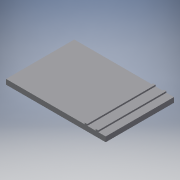
# Autodesk Inventor part: Zijkant 3
Saved by Autodesk Inventor 2018.3 (Build 223284000, 284)
## iProperties
Created: 2020-11-10
Part Number: Zijkant 3
Material: Generic
Document SubType Name: Modeling
Designer: daanv
Density: 1 g/cm^3
Appearance: Default
Author: daanv
Autodesk Inventor part; units mm, degrees
ref_plane "YZ Plane" through (0, 0, 0) normal (1, 0, 0) x (0, 1, 0)
ref_plane "XZ Plane" through (0, 0, 0) normal (0, 1, 0) x (-1, 0, 0)
ref_plane "XY Plane" through (0, 0, 0) normal (0, 0, 1) x (1, 0, 0)
sketch "Sketch1" plane through (0, 0, 0) normal (0, 0, 1) x (1, 0, 0)
  line L0 (0, 0) -> (20, 0)
  line L1 (20, 0) -> (20, 13.7)
  line L2 (20, 13.7) -> (0, 13.7)
  line L3 (0, 13.7) -> (0, 0)
  dimension "d0" = 20
  dimension "d1" = 13.7
  constraints: 8 end point, 2 parallel, 1 horizontal, 1 perpendicular
  measures "d0" distance of L2.end L1.end
  measures "d1" distance of L1.end L0.end
extrude "Extrusion1" add sketch "Sketch1" along normal blind 1
sketch "Sketch2" plane through (0, 0, 1) normal (0, 0, 1) x (1, 0, 0)
  line L0 (0, 0) -> (20, 0) projected
  line L1 (20, 13.7) -> (0, 13.7) projected
  line L2 (13.7, 13.7) -> (12.7, 13.7)
  line L3 (12.7, 13.7) -> (12.7, 0)
  line L4 (12.7, 0) -> (13.7, 0)
  line L5 (13.7, 0) -> (13.7, 13.7)
  line L6 (15.5, 0) -> (16.5, 0)
  line L7 (16.5, 0) -> (16.5, 13.7)
  line L8 (16.5, 13.7) -> (15.5, 13.7)
  line L9 (15.5, 13.7) -> (15.5, 0)
  dimension "d4" = 1
  dimension "d5" = 1
  dimension "d6" = 1.8
  dimension "d9" = 3.5
  constraints: 16 end point, 4 parallel, 4 point on line, 2 horizontal, 2 perpendicular
  measures "d4" distance of L4.end L3.end
  measures "d5" distance of L8.end L7.end
  measures "d6" distance of L8.end L2.start
  measures "d9" distance of L1.start L7.end
extrude "Extrusion2" add sketch "Sketch2" along normal blind 0.8 contours L3 L1 L5 L0 | L9 L1 L7 L0
body "Solid1"
